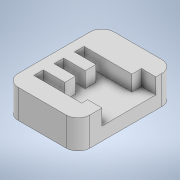
# Autodesk Inventor part: wooden_limitswitch
Saved by Autodesk Inventor 2020 (Build 240168000, 168)
## iProperties
Created: 2019-07-29
Part Number: wooden_limitswitch
Material: Generic
Document SubType Name: Modeling
Designer: erwin
Density: 1 g/cm^3
Appearance: Default
Author: erwin
Autodesk Inventor part; units mm, degrees
ref_plane "YZ Plane" through (0, 0, 0) normal (1, 0, 0) x (0, 1, 0)
ref_plane "XZ Plane" through (0, 0, 0) normal (0, 1, 0) x (-1, 0, 0)
ref_plane "XY Plane" through (0, 0, 0) normal (0, 0, 1) x (1, 0, 0)
sketch "Sketch1" plane through (0, 0, 0) normal (0, 1, 0) x (-1, 0, 0)
  line L0 (15, 20) -> (-15, 20)
  line L1 (-15, 20) -> (-15, -20)
  line L2 (-15, -20) -> (15, -20)
  line L3 (15, -20) -> (15, 20)
  line L4 (15, 20) -> (-15, -20) construction
  line L5 (-15, 20) -> (15, -20) construction
  point P0 (0, 0)
  dimension "d0" = 30
  dimension "d1" = 40
  constraints: 12 end point, 2 midpoint, 2 parallel, 1 horizontal, 1 perpendicular
  measures "d0" distance of L2.end L1.end
  measures "d1" distance of L1.end L0.end
extrude "Extrusion1" add sketch "Sketch1" along normal blind 12
sketch "Sketch2" plane through (0, 12, 0) normal (0, 1, 0) x (1, 0, 0)
  line L0 (15, -20) -> (15, 20) projected
  line L1 (15, -12.5) -> (-2, -12.5)
  line L2 (-2, 8.5) -> (9, 8.5)
  line L3 (15, 8.5) -> (15, -12.5)
  line L4 (15, -10) -> (9, -10)
  line L5 (9, -10) -> (9, -12.5)
  line L6 (9, -12.5) -> (15, -12.5)
  line L7 (15, -12.5) -> (15, -10)
  line L8 (-2, -12.5) -> (-7, -12.5)
  line L9 (-7, -12.5) -> (-7, -8.5)
  line L10 (-7, -8.5) -> (-2, -8.5)
  line L11 (-2, -8.5) -> (-2, -12.5)
  line L12 (-2, -4) -> (-7, -4)
  line L13 (-7, -4) -> (-7, 0)
  line L14 (-7, 0) -> (-2, 0)
  line L15 (-2, 8.5) -> (-7, 8.5)
  line L16 (-7, 8.5) -> (-7, 4.5)
  line L17 (-7, 4.5) -> (-2, 4.5)
  line L18 (-2, 4.5) -> (-2, 8.5)
  line L19 (15, 8.5) -> (9, 8.5)
  line L20 (9, 8.5) -> (9, 12.5)
  line L21 (9, 12.5) -> (15, 12.5)
  line L22 (15, 12.5) -> (15, 8.5)
  line L23 (-2, -8.5) -> (-2, -4)
  line L24 (-2, 0) -> (-2, 4.5)
  line L25 (-15, -20) -> (15, -20) projected
  line L26 (15, 20) -> (-15, 20) projected
  point P0 (0, 0)
  point P1 (15, -10)
  dimension "d4" = 21
  dimension "d5" = 17
  dimension "d7" = 2.5
  dimension "d8" = 5
  dimension "d9" = 4
  dimension "d10" = 4
  dimension "d11" = 4
  dimension "d12" = 4.5
  dimension "d13" = 4.5
  dimension "d14" = 4
  dimension "d15" = 7.5
  dimension "d22" = 25
  dimension "d23" = 7.5
  constraints: 48 end point, 12 parallel, 7 perpendicular, 6 horizontal, 5 point on line
  measures "d4" distance of L1.end L2.start
  measures "d5" distance of L1.start L1.end
  measures "d7" distance of L4.end L5.end
  measures "d8" distance of L10.end L9.end
  measures "d9" distance of L8.end L9.end
  measures "d10" distance of L15.end L16.end
  measures "d11" distance of L12.end L13.end
  measures "d12" distance between parallel lines of L17 L14
  measures "d13" distance between parallel lines of L12 L10
  measures "d14" distance of L2.end L20.end
  measures "d15" distance between parallel lines of L25 L1
  measures "d22" distance between parallel lines of L1 L21
  measures "d23" distance between parallel lines of L26 L21
extrude "Extrusion2" cut sketch "Sketch2" against normal blind 6.5 contours L4 L5 L1 L11 L23 L12 L13 L14 L24 L18 L2 L19 L0 | L19 L20 L21 L0 | L8 L9 L10 L11 | L18 L17 L16 L15
move faces "Move1" translate (-4, 0, 0) faces at (-7, 9.8333, 9.8333) (-7, 9.8333, 1.3333) (-7, 9.8333, -7.1667)
fillet "Fillet1" radius 5 4 edges at (-15, 6, -20) (-15, 6, 20) (15, 6, -20) (15, 6, 20)
equation "\"d10\" = d9"
equation "\"d11\" = d9"
equation "\"d13\" = d12"
equation "\"d15\" = d23"
body "Solid1"
